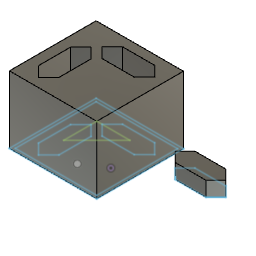
clock v2 (Autodesk Fusion 360 design; units mm, degrees)
Autodesk Fusion 360 part; units mm, degrees
sketch "Sketch1" plane through (0, 0, 0) normal (0, 0, 1) x (1, 0, 0)
  line L0 (-16.3137, 11.5) -> (-5, 11.5)
  line L1 (-5, 11.5) -> (-16.3137, 0.1863)
  line L2 (-16.3137, 0.1863) -> (-16.3137, 11.5)
  line L3 (-14.5, 11.5) -> (-11, 15)
  line L4 (-11, 15) -> (0, 15)
  line L5 (0, 15) -> (3.5, 11.5)
  line L6 (3.5, 11.5) -> (0, 8)
  line L7 (0, 8) -> (-11, 8)
  line L8 (-11, 8) -> (-14.5, 11.5)
  line L9 (-19.8, 6) -> (-16.3, 9.5)
  line L10 (-12.8, -5) -> (-16.3, -8.5)
  line L11 (-16.3, 9.5) -> (-12.8, 6)
  line L12 (-19.8, -5) -> (-19.8, 6)
  line L13 (-16.3, -8.5) -> (-19.8, -5)
  line L14 (-12.8, 6) -> (-12.8, -5)
  line L15 (-23.2399, 18.1875) -> (6.6848, 18.1875)
  line L16 (6.6848, 18.1875) -> (6.6848, -11.5279)
  line L17 (6.6848, -11.5279) -> (-23.2399, -11.5279)
  line L18 (-23.2399, -11.5279) -> (-23.2399, 18.1875)
  line L19 (-22.2399, 17.1875) -> (5.6848, 17.1875)
  line L20 (5.6848, 17.1875) -> (5.6848, -10.5279)
  line L21 (5.6848, -10.5279) -> (-22.2399, -10.5279)
  line L22 (-22.2399, -10.5279) -> (-22.2399, 17.1875)
  line L23 (11.04, 11.04) -> (14.4, 14.4)
  line L24 (14.4, 7.68) -> (11.04, 11.04)
  line L25 (24.96, 7.68) -> (14.4, 7.68)
  line L26 (28.32, 11.04) -> (24.96, 7.68)
  line L27 (24.96, 14.4) -> (28.32, 11.04)
  line L28 (14.4, 14.4) -> (24.96, 14.4)
  point P0 (-7, -4.5)
  dimension "d3" = 11.3137
  dimension "d11" = 7
  dimension "d14" = 18
  dimension "d21" = 1
  dimension "d22" = 1
  dimension "d23" = 1
  dimension "d24" = 1
  constraint horizontal L0
  constraint perpendicular L0 L2
  constraint horizontal L4
  constraint perpendicular L3 L5
  constraint perpendicular L5 L6
  constraint parallel L4 L7
  constraint perpendicular L3 L8
  constraint equal L5 L6
  constraint equal L3 L8
  constraint horizontal L15
  constraint vertical L16
  constraint horizontal L17
  constraint vertical L18
  constraint horizontal L19
  constraint vertical L20
  constraint horizontal L21
  constraint vertical L22
  constraint horizontal L28
  constraint perpendicular L23 L27
  constraint perpendicular L26 L27
  constraint parallel L25 L28
  constraint perpendicular L23 L24
  constraint equal L26 L27
  constraint equal L23 L24
  measures "d3" distance of L0.start L1.end
  measures "d11" distance of L4 L7
  measures "d14" distance of L3.start L5.end
  measures "d21" distance of L15 L19
  measures "d22" distance of L16 L20
  measures "d23" distance of L17 L21
  measures "d24" distance of L18 L22
extrude "Extrude2" add sketch "Sketch1" along normal blind 23 contours L0 L1 L2 L7 L8 L9 L11 L14 | L15 L16 L17 L18 | L19 L20 L21 L22 makes body 1
extrude "Extrude3" cut sketch "Sketch1" along normal blind 16 contours L0 L1 L2 L7 L8 L9 L11 L14 | L0 L1 L3 L4 L5 L6 L7 | L0 L1 L7 L8 | L1 L2 L9 L11 L14 | L1 L2 L9 L10 L12 L13 L14 | L19 L20 L21 L22 bodies 1
extrude "Extrude4" add sketch "Sketch1" along normal blind 5 separate body contours L23 L24 L25 L26 L27 L28 makes body 2
equation "vspace = 11.313708499 mm"
equation "d11 = thickboy"
equation "thickboy = 7 mm"
equation "with = 18 mm"
equation "d14 = with"
equation "tol = 0.127 mm"
